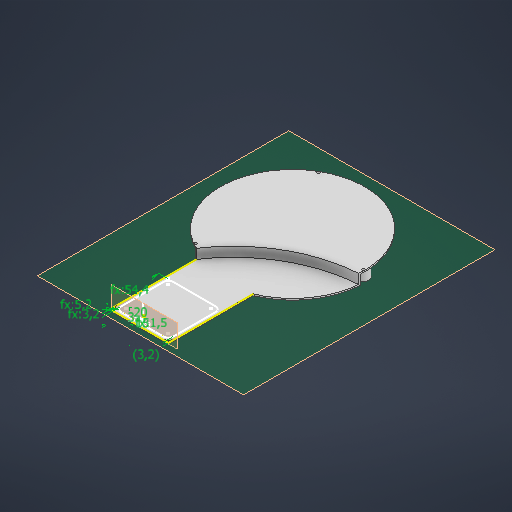
# Autodesk Inventor part: bottom_replacement_housing_bottom
Saved by Autodesk Inventor 2026 (Build 300175000, 175)
## iProperties
Created: 2025-05-12
Part Number: bottom_replacement_housing_bottom
Material: Generic
Document SubType Name: Sheet Metal
Designer: Paul Juschitz
Density: 1 g/cm^3
Sheet Metal Rule: Default_mm
Appearance: Default
d0: 1,000 ul
bottom_screwhole_diameter: 2,500 mm
bottom_screwhole_spacing: 128,000 mm
bottom_screwhole_angle: 30,00 deg
d6: 150,600 mm
bottom_material_thickness: 1,500 mm
d8: 0,00 deg
bottom_cutout_radius: 140,000 mm
bottom_cutout_angle: 120,00 deg
bottom_cutout_clearance: 5,000 mm
d13: 0,00 deg
d16: 1,500 mm
bottom_extension__height: 10,000 mm
d18: 0,00 deg
d19: -1,500 mm
bottom_extension_outset: 90,000 mm
bottom_core_outer_width: 60,800 mm
d27: 0,00 deg
bottom_foot_OD: 12,500 mm
bottom_foot_inset: 2,000 mm
d30: 2,000 mm
d31: 5,000 ul
bottom_foot_height: 11,000 mm
d36: 0,00 deg
d37: 1,000 mm
d38: 1,000 mm
d39: 0,00 deg
d41: 0,00 deg
d46: 0,00 deg
d47: 25,000 mm
d49: 0,00 deg
d51: 0,00 deg
d33: 360,00 deg
m2m_shell_bottom_screwhole_inset: -2,000 mm
m2m_shell_bottom_screwhole_ID: 2,500 mm
m2m_shell_bottom_screwhole_OD: 3,900 mm
m2m_bottom_radius_lower: 76,000 mm
m2m_bottom_radius_upper: 68,000 mm
m2m_shell_thickness: 0,500 mm
m2m_shell_height: 220,000 mm
m2m_shell_base_height: 16,000 mm
bottom_distance_tolerance: 0,200 mm
bottom_lip_height: 5,000 mm
core_outer_width: 54,000 mm
core_outer_radius: 5,000 mm
core_height: 25,000 mm
Author: Paul Juschitz
Autodesk Inventor part; units mm, degrees
ref_plane "YZ Plane" through (0, 0, 0) normal (1, 0, 0) x (0, 1, 0)
ref_plane "XZ Plane" through (0, 0, 0) normal (0, 1, 0) x (-1, 0, 0)
derived "m2m_shell.ipt"
sketch "Sketch1" plane through (0, 0, 0) normal (0, 1, 0) x (-1, 0, 0)
  circle A0 centre (36.9504, 64) radius 1.25
  circle A1 centre (36.9504, -64) radius 1.25
  circle A2 centre (-73.9008, 0) radius 1.25
  line L0 (36.9504, 64) -> (36.9504, -64) construction
  line L1 (36.9504, -64) -> (-73.9008, 0) construction
  line L2 (-73.9008, 0) -> (36.9504, 64) construction
  line L3 (-73.9008, 0) -> (36.9504, 0)
  line L4 (36.9504, 64) -> (-18.4752, -32)
  line L5 (36.9504, -64) -> (-18.4752, 32)
  line L6 (0, -136.5769) -> (0, 186.0374) construction
  circle A3 centre (0, 0) radius 75.3
  dimension "bottom_screwhole_diameter" = 2.5
  dimension "bottom_screwhole_spacing" = 128
  dimension "bottom_screwhole_angle" = 30
  dimension "d6" = 150.6
  constraints: 14 end point, 4 centre point, 3 midpoint, 2 coincident, 2 equal length, 2 equal radius, 2 point on line, 1 vertical, 2 other
  measures "bottom_screwhole_diameter" diameter of A0
  measures "bottom_screwhole_spacing" distance of L0.end L1.end
  measures "bottom_screwhole_angle" angle of L6 L5
  measures "d6" diameter of A3
extrude "Extrusion1" add sketch "Sketch1" along normal blind 1.5
sketch "Sketch2" plane through (0, 1.5, 0) normal (0, 1, 0) x (1, 0, 0)
  circle A0 centre (0, 0) radius 75.3 construction
  arc A1 (75.0454, -6.1864) -> (-32.1651, -68.0845) centre (84.2268, -145.885) ccw
  line L0 (-75.3, 0) -> (75.3, 0) construction
  line L1 (84.2268, -145.885) -> (0, 0) construction
  circle A2 centre (-36.9504, -64) radius 1.25 projected
  arc A3 (-32.1651, -68.0845) -> (75.0454, -6.1864) centre (0, 0) ccw
  dimension "bottom_cutout_radius" = 140
  dimension "bottom_cutout_angle" = 120
  dimension "bottom_cutout_clearance" = 5
  constraints: 10 point on circle, 4 end point, 2 centre point, 1 concentric, 1 horizontal, 1 line through centre
  measures "bottom_cutout_radius" radius of A1
  measures "bottom_cutout_angle" angle of L0 L1
extrude "Extrusion2" cut sketch "Sketch2" against normal through all contours A3 A1
sketch "Sketch3" plane through (0, 0, 0) normal (0, -1, 0) x (1, 0, 0)
  arc A0 (-32.1651, 68.0845) -> (75.0454, 6.1864) centre (84.2268, 145.885) ccw projected
  arc A1 (-32.1651, 68.0845) -> (75.0454, 6.1864) centre (0, 0) ccw construction
  circle A2 centre (73.9008, 0) radius 1.25 construction
  circle A3 centre (-36.9504, 64) radius 1.25 construction
  arc A4 (75.1547, 4.6761) -> (75.0454, 6.1864) centre (0, 0) ccw
  arc A5 (-33.5277, 67.4239) -> (75.1547, 4.6761) centre (84.2268, 145.885) ccw
  arc A6 (-32.1651, 68.0845) -> (-33.5277, 67.4239) centre (0, 0) ccw
  dimension "d16" = 1.5
  constraints: 8 point on circle, 3 centre point, 3 coincident
  measures "d16" radial gap between concentric circles of A5 A0
extrude "Extrusion3" add sketch "Sketch3" along normal blind 10
ref_plane "bottom extension plane" through (0, -8.5, 0) normal (0, -1, 0) x (1, 0, 0)
sketch "Sketch4" plane through (0, -8.5, 0) normal (0, -1, 0) x (1, 0, 0)
  arc A0 (-32.1651, 68.0845) -> (75.0454, 6.1864) centre (84.2268, 145.885) ccw projected
  arc A1 (-32.1651, 68.0845) -> (75.0454, 6.1864) centre (0, 0) ccw construction
  circle A2 centre (0, 0) radius 75.3 construction
  line L0 (-32.1651, 68.0845) -> (-32.1651, 158.0845)
  line L1 (-32.1651, 158.0845) -> (28.6349, 158.0845)
  line L2 (28.6349, 158.0845) -> (28.6349, 69.6429)
  arc A3 (75.0454, 6.1864) -> (28.6349, 69.6429) centre (0, 0) ccw
  dimension "bottom_extension_outset" = 90
  dimension "bottom_core_outer_width" = 60.8
  constraints: 6 end point, 2 perpendicular, 2 point on circle, 1 centre point, 1 concentric, 1 vertical, 6 other
  measures "bottom_extension_outset" distance of L0.start L0.end
  measures "bottom_core_outer_width" distance of L0.end L1.end
extrude "Extrusion5" add sketch "Sketch4" along normal up to surface (1.5 mm away)
sketch "Sketch5" plane through (0, 0, 0) normal (0, -1, 0) x (1, 0, 0)
  arc A0 (-33.5277, 67.4239) -> (75.1547, 4.6761) centre (0, 0) ccw construction
  circle A1 centre (66.7569, -6.2622) radius 6.25
  circle A2 centre (73.9008, 0) radius 1.25 projected
  circle A3 centre (26.5847, 61.5545) radius 6.25
  circle A4 centre (-50.3267, 44.3049) radius 6.25
  circle A5 centre (-57.6883, -34.1725) radius 6.25
  circle A6 centre (14.6734, -65.4247) radius 6.25
  dimension "bottom_foot_OD" = 12.5
  dimension "bottom_foot_inset" = 2
  dimension "d30" = 2
  dimension "d33" = 360
  constraints: 5 centre point, 1 coincident, 11 other
  measures "bottom_foot_OD" diameter of A1
extrude "Extrusion6" add sketch "Sketch5" along normal blind 11 contours A1 | A4 | A5 | A6
sketch "Sketch6" plane through (66.7569, -11, -6.2622) normal (0, -1, 0) x (1, 0, 0)
  circle A0 centre (0, 0) radius 6.25 projected
  circle A1 centre (-52.0836, -59.1626) radius 6.25 projected
  circle A2 centre (-124.4452, -27.9104) radius 6.25 projected
  circle A3 centre (-117.0836, 50.5671) radius 6.25 projected
  circle A4 centre (0, 0) radius 5.25
  circle A5 centre (-52.0836, -59.1626) radius 5.25
  circle A6 centre (-124.4452, -27.9104) radius 5.25
  circle A7 centre (-117.0836, 50.5671) radius 5.25
  point P0 (-66.7569, 6.2622)
  dimension "d37" = 1
  constraints: 4 centre point, 4 coincident, 3 equal radius
  measures "d37" radial gap between concentric circles of A3 A7
extrude "Extrusion7" add sketch "Sketch6" along normal blind 1
sketch "Sketch7" plane through (0, -10, 0) normal (0, -1, 0) x (1, 0, 0)
  circle A0 centre (26.5847, 61.5545) radius 6.25 projected
  point P0 (0, 0)
extrude "Extrusion8" add sketch "Sketch7" along normal up to surface (2 mm away)
sketch "Sketch10" plane through (26.5847, -12, 61.5545) normal (0, -1, 0) x (1, 0, 0)
  circle A0 centre (0, 0) radius 6.25 construction
  circle A1 centre (40.1722, -67.8167) radius 5.25 construction
  circle A2 centre (0, 0) radius 5.25
  point P0 (-26.5847, -61.5545)
  constraints: 1 centre point, 1 coincident, 1 equal radius
extrude "Extrusion10" cut sketch "Sketch10" against normal up to surface (1 mm away)
sketch "Sketch11" plane through (0, -10, 0) normal (0, -1, 0) x (1, 0, 0)
  line L0 (-32.1651, 158.0845) -> (28.6349, 158.0845) construction
  line L1 (28.6349, 158.0845) -> (28.6349, 69.6429) construction
  line L2 (-32.1651, 68.0845) -> (-32.1651, 158.0845) construction
  circle A0 centre (26.5847, 61.5545) radius 6.25 construction
  circle A1 centre (26.5847, 61.5545) radius 5.25 construction
  line L3 (-1.7651, 158.0845) -> (-1.7651, 33.5122)
  arc A2 (-33.5277, 67.4239) -> (75.1547, 4.6761) centre (84.2268, 145.885) ccw projected
  circle A3 centre (-1.7651, 133.0845) radius 6.25
  circle A4 centre (-1.7651, 133.0845) radius 5.25
  point P0 (0, 0)
  dimension "d47" = 25
  constraints: 2 centre point, 2 end point, 2 equal radius, 1 coincident, 1 midpoint, 1 point on circle, 1 point on line, 1 vertical
  measures "d47" distance from line of L0 A3.centre
extrude "Extrusion11" add sketch "Sketch11" along normal up to surface (2 mm away) contours A3 L3 A4 | L3 A4 A3
sketch "Sketch12" plane through (-1.7651, -10, 133.0845) normal (0, -1, 0) x (1, 0, 0)
  circle A0 centre (0, 0) radius 5.25 projected
  point P0 (1.7651, -133.0845)
extrude "Extrusion12" add sketch "Sketch12" along normal up to surface (1 mm away)
derived "core_dummy.ipt"
ref_plane "Floor" through (66.7569, -12, -6.2622) normal (0, -1, 0) x (1, 0, 0)
sketch "Sketch13" plane through (0, -8.5, 0) normal (0, 1, 0) x (1, 0, 0)
  line L0 (-23.7651, -154.8845) -> (20.2349, -154.8845)
  line L1 (25.4349, -149.6845) -> (25.4349, -105.6845)
  line L2 (20.2349, -100.4845) -> (-23.7651, -100.4845)
  line L3 (-28.9651, -105.6845) -> (-28.9651, -149.6845)
  line L4 (-32.1651, -158.0845) -> (-32.1651, -68.0845) projected
  line L5 (25.4349, -154.8845) -> (25.4349, -158.0845) construction
  line L6 (-32.1651, -158.0845) -> (28.6349, -158.0845) projected
  line L7 (-28.9651, -154.8845) -> (-32.1651, -154.8845) construction
  arc A0 (-28.9651, -149.6845) -> (-23.7651, -154.8845) centre (-23.7651, -149.6845) ccw
  arc A1 (20.2349, -154.8845) -> (25.4349, -149.6845) centre (20.2349, -149.6845) ccw
  arc A2 (25.4349, -105.6845) -> (20.2349, -100.4845) centre (20.2349, -105.6845) ccw
  arc A3 (-23.7651, -100.4845) -> (-28.9651, -105.6845) centre (-23.7651, -105.6845) ccw
  line L8 (28.6349, -69.6429) -> (28.6349, -158.0845) projected
  point P0 (0, 0)
  point P1 (-28.9651, -100.4845)
  dimension "d54" = 3.2
  dimension "d56" = 54.4
  dimension "d57" = 5.2
  dimension "d59" = 3.2
  constraints: 12 end point, 8 point on circle, 8 point on line, 8 tangent, 4 centre point, 4 perpendicular, 3 equal radius, 2 parallel, 1 horizontal, 1 vertical
  measures "d54" distance between parallel lines of L4 L3
  measures "d56" distance of point (-28.965, -100.484) L7.start
  measures "d57" radius of A0
  measures "d59" distance between parallel lines of L8 L1
fillet "Fillet1" radius 8.2 2 edges at (28.6349, -9.25, 158.0845) (-32.1651, -9.25, 158.0845)
ref_plane "Work Plane3" through (-23.7651, -8.5, 154.8845) normal (0, 0, 1) x (1, 0, 0)
sketch "Sketch14" plane through (-23.7651, -8.5, 154.8845) normal (0, 0, 1) x (1, 0, 0)
  line L0 (0, 0) -> (44, 0) construction
  line L1 (22, 0) -> (22, 20)
  line L2 (14.5, 4.5) -> (29.5, 4.5)
  line L3 (29.5, 4.5) -> (29.5, 3)
  line L4 (29.5, 3) -> (14.5, 3)
  line L5 (14.5, 3) -> (14.5, 4.5)
  line L6 (14.5, 4.5) -> (29.5, 3) construction
  line L7 (29.5, 4.5) -> (14.5, 3) construction
  point P0 (23.7651, 8.5)
  point P1 (22, 3.75)
  dimension "d61" = 20
  dimension "bottom_connector_lip_width" = 15
  dimension "d63" = 1.5
  dimension "bottom_connector_lip_height" = 3
  constraints: 14 end point, 3 midpoint, 2 parallel, 1 horizontal, 1 perpendicular, 1 point on line, 1 vertical
  measures "d61" distance of L1.start L1.end
  measures "bottom_connector_lip_width" distance of L3.end L4.end
  measures "d63" distance of L2.end L3.end
  measures "bottom_connector_lip_height" distance from line of L0 L4.end
equation "\"bottom_screwhole_diameter\" = m2m_shell_bottom_screwhole_ID"
equation "\"d6\" = -2 * bottom_distance_tolerance + 2 * m2m_bottom_radius_lower - 2 * m2m_shell_thickness"
equation "\"d16\" = bottom_material_thickness"
equation "\"bottom_core_outer_width\" = 4 * bottom_distance_tolerance + core_outer_width + 4 * bottom_material_thickness"
equation "\"d54\" = 2 * bottom_material_thickness + bottom_distance_tolerance"
equation "\"d56\" = core_outer_width + 2 * bottom_distance_tolerance"
equation "\"d57\" = core_outer_radius + bottom_distance_tolerance"
equation "\"d58\" = bottom_distance_tolerance + core_outer_radius + 2 * bottom_material_thickness"
equation "\"d63\" = bottom_material_thickness"
equation "\"BendRadius\" = Thickness"
equation "\"BendReliefWidth\" = Thickness"
equation "\"BendReliefDepth\" = 0.5 * Thickness"
equation "\"CornerReliefSize\" = 4 * Thickness"
equation "\"MinimumRemnant\" = 2 * Thickness"
equation "\"TransitionRadius\" = BendRadius"
equation "\"JacobiRadiusSize\" = BendRadius"
equation "\"GapSize\" = Thickness"
equation "\"d19\" = -bottom_material_thickness"
equation "\"bottom_distance_tolerance\" = 0.2"
equation "\"bottom_lip_height\" = 5"
equation "\"m2m_shell_bottom_screwhole_ID\" = 2.5"
equation "\"m2m_bottom_radius_lower\" = 76"
equation "\"m2m_shell_thickness\" = 0.5"
equation "\"bottom_material_thickness\" = 1.5"
equation "\"core_outer_width\" = 54"
equation "\"core_outer_radius\" = 5"
equation "\"Thickness\" = 0.5"
body "Solid1"
